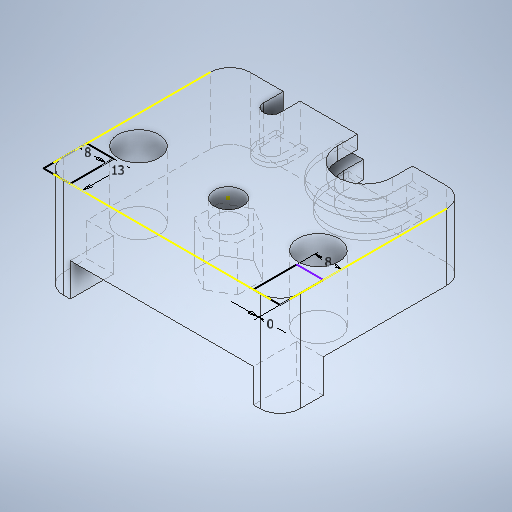
# Autodesk Inventor part: Guideteil_Spritzenpumpe001
Saved by Autodesk Inventor 2025 (Build 290162000, 162)
## iProperties
Created: 2024-04-11
Part Number: Guideteil_Spritzenpumpe001
Material: Generisch
Document SubType Name: Modeling
Designer: noahm
Density: 1 g/cm^3
Appearance: Vorgabe
Author: noahm
Autodesk Inventor part; units mm, degrees
ref_plane "YZ Plane" through (0, 0, 0) normal (1, 0, 0) x (0, 1, 0)
ref_plane "XZ Plane" through (0, 0, 0) normal (0, 1, 0) x (-1, 0, 0)
ref_plane "XY Plane" through (0, 0, 0) normal (0, 0, 1) x (1, 0, 0)
sketch "Skizze1" plane through (0, 0, 0) normal (0, 0, 1) x (1, 0, 0)
  line L0 (-35.5, 36) -> (35.5, 36)
  line L1 (35.5, 36) -> (35.5, -20)
  line L2 (35.5, -20) -> (-35.5, -20)
  line L3 (-35.5, -20) -> (-35.5, 36)
  circle A0 centre (0, 0) radius 4.25
  circle A1 centre (-27, 0) radius 6.125
  circle A2 centre (27, 0) radius 6.125
  point P0 (0, -20)
  point P1 (35.5, 8)
  dimension "d0" = 71
  dimension "d1" = 56
  dimension "d2" = 20
  dimension "d3" = 35.5
  dimension "d4" = 8.5
  dimension "d5" = 12.25
  dimension "d6" = 12.25
  dimension "d7" = 27
  dimension "d8" = 27
  constraints: 8 end point, 3 centre point, 2 midpoint, 2 parallel, 1 coincident, 1 horizontal, 1 perpendicular
  measures "d0" distance of L0.start L0.end
  measures "d1" distance of L2.end L0.start
  measures "d2" distance of point (0, 0) point (0, -20)
  measures "d3" horizontal distance of point (0, 0) point (35.5, 8)
  measures "d4" diameter of A0
  measures "d5" diameter of A1
  measures "d6" diameter of A2
  measures "d7" distance of point (0, 0) A2.centre
  measures "d8" distance of point (0, 0) A1.centre
extrude "Extrusion1" add sketch "Skizze1" along normal blind 9
sketch "Skizze2" plane through (0, 0, 9) normal (0, 0, 1) x (1, 0, 0)
  arc A0 (-22.5, 30) -> (-11.5, 30) centre (-17, 30) ccw
  arc A1 (0, 30) -> (22, 30) centre (11, 30) ccw
  line L0 (35.5, 36) -> (-35.5, 36) projected
  line L1 (-35.5, 36) -> (-35.5, -20) projected
  line L2 (35.5, -20) -> (35.5, 36) projected
  line L3 (-22.5, 30) -> (-22.5, 36)
  line L4 (-11.5, 30) -> (-11.5, 36)
  line L5 (0, 30) -> (0, 36)
  line L6 (22, 30) -> (22, 36)
  point P0 (0, 0)
  dimension "d11" = 11
  dimension "d12" = 22
  dimension "d13" = 6
  dimension "d14" = 6
  dimension "d15" = 18.5
  dimension "d16" = 24.5
  constraints: 8 end point, 4 point on circle, 3 perpendicular, 3 point on line, 3 tangent, 2 centre point, 1 midpoint
  measures "d11" diameter of A0
  measures "d12" diameter of A1
  measures "d13" distance from line of L0 A0.centre
  measures "d14" distance from line of L0 A1.centre
  measures "d15" distance from line of L1 A0.centre
  measures "d16" distance from line of L2 A1.centre
extrude "Extrusion2" cut sketch "Skizze2" against normal blind 1.67
sketch "Skizze3" plane through (0, 0, 9) normal (0, 0, 1) x (1, 0, 0)
  line L0 (-22.5, 36) -> (-35.5, 36) projected
  line L1 (35.5, 36) -> (35.5, -20)
  line L2 (35.5, -20) -> (-35.5, -20)
  line L3 (-35.5, -20) -> (-35.5, 36)
  circle A0 centre (-27, 0) radius 6.125
  circle A1 centre (0, 0) radius 4.25
  circle A2 centre (27, 0) radius 6.125
  circle A3 centre (27, 0) radius 6.125 projected
  circle A4 centre (-27, 0) radius 6.125 projected
  arc A5 (-19.5, 30) -> (-14.5, 30) centre (-17, 30) ccw
  arc A6 (-22.5, 30) -> (-11.5, 30) centre (-17, 30) ccw projected
  arc A7 (4.5, 30) -> (17.5, 30) centre (11, 30) ccw
  arc A8 (0, 30) -> (22, 30) centre (11, 30) ccw projected
  line L4 (-19.5, 30) -> (-19.5, 36)
  line L5 (-14.5, 30) -> (-14.5, 36)
  line L6 (4.5, 30) -> (4.5, 36)
  line L7 (17.5, 30) -> (17.5, 36)
  line L8 (17.5, 36) -> (35.5, 36)
  line L9 (-35.5, 36) -> (-19.5, 36)
  line L10 (-14.5, 36) -> (4.5, 36)
  dimension "d19" = 71
  dimension "d20" = 56
  dimension "d21" = 12.25
  dimension "d22" = 12.25
  dimension "d23" = 0
  dimension "d24" = 0
  dimension "d25" = 5
  dimension "d26" = 0
  dimension "d27" = 13
  dimension "d28" = 0
  dimension "d29" = 0
  dimension "d30" = 0
  constraints: 20 end point, 17 perpendicular, 5 centre point, 4 point on circle, 3 collinear, 3 tangent, 1 coincident
  measures "d19" distance of L0.end L1.start
  measures "d20" distance of L1.start L1.end
  measures "d21" diameter of A0
  measures "d22" diameter of A2
  measures "d23" radial gap between concentric circles of A3 A2
  measures "d24" distance of A4.centre A0.centre
  measures "d25" diameter of A5
  measures "d26" distance of A6.centre A5.centre
  measures "d27" diameter of A7
  measures "d28" distance of A8.centre A7.centre
  measures "d29" distance of A8.centre A7.centre
  measures "d30" distance of A6.centre A5.centre
extrude "Extrusion3" add sketch "Skizze3" along normal blind 11
fillet "Rundung1" radius 6 2 edges at (35.5, 36, 10) (-35.5, 36, 10)
fillet "Rundung2" radius 3 2 edges at (-35.5, -20, 10) (35.5, -20, 10)
sketch "Skizze4" plane through (0, 0, 20) normal (0, 0, 1) x (1, 0, 0)
  line L0 (-32.5, -20) -> (32.5, -20) projected
  line L1 (-35.5, 30) -> (-35.5, -17) projected
  line L2 (-27.5, -20) -> (-35.5, -20)
  line L3 (-35.5, -20) -> (-35.5, -7)
  line L4 (-35.5, -7) -> (-27.5, -7)
  line L5 (-27.5, -7) -> (-27.5, -20)
  line L6 (27.5, -20) -> (35.5, -20)
  line L7 (35.5, -20) -> (35.5, -7)
  line L8 (35.5, -7) -> (27.5, -7)
  line L9 (27.5, -7) -> (27.5, -20)
  line L10 (35.5, -17) -> (35.5, 30) projected
  point P0 (0, 0)
  point P1 (-35.5, -17)
  dimension "d35" = 8
  dimension "d36" = 13
  dimension "d37" = 8
  dimension "d38" = 0
  constraints: 16 end point, 4 parallel, 3 point on line, 2 horizontal, 2 perpendicular
  measures "d35" distance of L3.end L4.end
  measures "d36" distance of L4.end L2.start
  measures "d37" distance of L8.end L7.end
  measures "d38" distance between parallel lines of L10 L7
sketch "Skizze5" plane through (0, 0, 0) normal (0, 0, -1) x (-1, 0, 0)
  line L0 (32.5, -20) -> (-32.5, -20) projected
  line L1 (35.5, 30) -> (35.5, -17) projected
  line L2 (27.5, -20) -> (35.5, -20)
  line L3 (35.5, -20) -> (35.5, -7)
  line L4 (35.5, -7) -> (27.5, -7)
  line L5 (27.5, -7) -> (27.5, -20)
  line L6 (-35.5, -14) -> (-35.5, -7) projected
  line L7 (-35.5, -7) -> (-27.5, -7)
  line L8 (-27.5, -7) -> (-27.5, -20)
  line L9 (-27.5, -20) -> (-35.5, -20)
  line L10 (-35.5, -20) -> (-35.5, -7)
  point P0 (0, 0)
  point P1 (29.5, -20)
  point P2 (-29.5, -20)
  point P3 (35.5, -14)
  point P4 (29.5, -20)
  point P5 (35.5, -14)
  point P6 (-29.5, -20)
  dimension "d42" = 13
  dimension "d43" = 8
  dimension "d44" = 8
  constraints: 16 end point, 4 parallel, 3 point on line, 2 horizontal, 2 perpendicular
  measures "d42" distance of L4.end L2.start
  measures "d43" distance of L3.end L4.end
  measures "d44" distance of L8.end L9.end
extrude "Extrusion5" add sketch "Skizze5" along normal blind 10
fillet "Rundung4" radius 6 2 edges at (-35.5, -20, -5) (35.5, -20, -5)
sketch "Skizze6" plane through (0, 0, 0) normal (0, 0, -1) x (-1, 0, 0)
  line L0 (6.5705, -3.7459) -> (0.0412, -7.5632)
  line L1 (0.0412, -7.5632) -> (-6.5293, -3.8173)
  line L2 (-6.5293, -3.8173) -> (-6.5705, 3.7459)
  line L3 (-6.5705, 3.7459) -> (-0.0412, 7.5632)
  line L4 (-0.0412, 7.5632) -> (6.5293, 3.8173)
  line L5 (6.5293, 3.8173) -> (6.5705, -3.7459)
  point P0 (0, 0)
  point P1 (0, 0)
  point P2 (-6.5499, -0.0357)
  dimension "d48" = 13.1
  constraints: 12 end point, 1 coincident, 1 midpoint, 13 other
  measures "d48" distance from line of point (-6.55, -0.036) L5
extrude "Extrusion6" cut sketch "Skizze6" against normal blind 13.5
sketch "Skizze7" plane through (0, 0, 7.33) normal (0, 0, 1) x (1, 0, 0)
  arc A0 (-22.5, 30) -> (-11.5, 30) centre (-17, 30) ccw projected
  line L0 (-22.5, 30) -> (-22.5, 36) projected
  line L1 (-11.5, 36) -> (-11.5, 30) projected
  line L2 (-22.5, 36) -> (-11.5, 36) projected
  point P0 (0, 0)
extrude "Extrusion7" add sketch "Skizze7" along normal blind 0.4
sketch "Skizze8" plane through (0, 0, 7.73) normal (0, 0, 1) x (1, 0, 0)
  arc A0 (-22.5, 30) -> (-11.5, 30) centre (-17, 30) ccw projected
  arc A1 (-21.6, 30) -> (-12.4, 30) centre (-17, 30) ccw
  line L0 (-21.6, 30) -> (-21.6, 36)
  line L1 (-11.5, 36) -> (-22.5, 36) projected
  line L2 (-12.4, 30) -> (-12.4, 36)
  line L3 (-22.5, 30) -> (-22.5, 36) projected
  line L4 (-11.5, 36) -> (-11.5, 30) projected
  line L5 (4.5, 36) -> (-14.5, 36) projected
  line L6 (-19.5, 36) -> (-29.5, 36) projected
  point P0 (0, 0)
  dimension "d53" = 9.2
  constraints: 4 end point, 2 point on circle, 2 point on line, 1 centre point, 1 coincident, 1 parallel, 1 tangent, 1 vertical
  measures "d53" diameter of A1
extrude "Extrusion8" add sketch "Skizze8" along normal blind 1.27 contours L3 L1 L0 A1 L2 L4 A0
sketch "Skizze9" plane through (0, 0, 20) normal (0, 0, 1) x (1, 0, 0)
  arc A0 (0, 30) -> (22, 30) centre (11, 30) ccw projected
  line L0 (2.75, 30) -> (2.75, 36)
  line L1 (0, 36) -> (22, 36) projected
  line L2 (19.25, 30) -> (19.25, 36)
  arc A1 (2.75, 30) -> (19.25, 30) centre (11, 30) ccw
  point P0 (0, 0)
  constraints: 4 end point, 2 point on circle, 2 point on line, 1 centre point, 1 coincident, 1 parallel, 1 tangent, 1 vertical
extrude "Extrusion9" cut sketch "Skizze9" against normal blind 4
sketch "Skizze10" plane through (0, 0, 16) normal (0, 0, 1) x (1, 0, 0)
  arc A0 (0, 30) -> (22, 30) centre (11, 30) ccw projected
  line L0 (-1.8, 30) -> (-1.8, 36)
  line L1 (0, 36) -> (22, 36) projected
  line L2 (2.75, 36) -> (-14.5, 36) projected
  line L3 (29.5, 36) -> (19.25, 36) projected
  line L4 (23.8, 30) -> (23.8, 36)
  arc A1 (-1.8, 30) -> (23.8, 30) centre (11, 30) ccw
  point P0 (0, 0)
  constraints: 4 end point, 2 point on circle, 1 centre point, 1 coincident, 1 perpendicular, 1 point on line, 1 tangent, 1 vertical
extrude "Extrusion10" cut sketch "Skizze10" against normal blind 1.67
